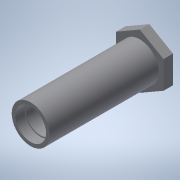
# Autodesk Inventor part: steering_stand_off_bush
Saved by Autodesk Inventor 2020 (Build 240168000, 168)
## iProperties
Created: 2015-12-06
Part Number: steering_stand_off_bush
Material: Genérico
Document SubType Name: Modeling
Designer: MIGUEL ANGEL
Density: 1 g/cm^3
Appearance: Valor por defecto
Author: MIGUEL ANGEL
Autodesk Inventor part; units mm, degrees
ref_plane "YZ Plane" through (0, 0, 0) normal (1, 0, 0) x (0, 1, 0)
ref_plane "XZ Plane" through (0, 0, 0) normal (0, 1, 0) x (-1, 0, 0)
ref_plane "XY Plane" through (0, 0, 0) normal (0, 0, 1) x (1, 0, 0)
sketch "Boceto1" plane through (0, 0, 0) normal (0, 1, 0) x (-1, 0, 0)
  circle A0 centre (0, 0) radius 8
  dimension "d0" = 16
  constraints: 1 centre point, 1 coincident
  measures "d0" diameter of A0
extrude "Extrusión1" add sketch "Boceto1" along normal blind 46
sketch "Boceto2" plane through (0, 46, 0) normal (0, 1, 0) x (1, 0, 0)
  line L0 (0, 11.547) -> (10, 5.7735)
  line L1 (10, 5.7735) -> (10, -5.7735)
  line L2 (10, -5.7735) -> (0, -11.547)
  line L3 (0, -11.547) -> (-10, -5.7735)
  line L4 (-10, -5.7735) -> (-10, 5.7735)
  line L5 (-10, 5.7735) -> (0, 11.547)
  point P0 (0, 0)
  point P1 (0, 0)
  point P2 (-10, 0)
  dimension "d3" = 10
  constraints: 12 end point, 1 coincident, 1 horizontal alignment, 1 midpoint, 13 other
  measures "d3" horizontal distance of L1.end L2.end
extrude "Extrusión2" add sketch "Boceto2" along normal blind 4
sketch "Boceto3" plane through (0, 0, 0) normal (0, -1, 0) x (1, 0, 0)
  circle A0 centre (0, 0) radius 8 projected
  circle A1 centre (0, 0) radius 6
  dimension "d6" = 2
  constraints: 1 centre point
  measures "d6" radial gap between concentric circles of A0 A1
extrude "Extrusión3" cut sketch "Boceto3" against normal through all contours A1
sketch "Boceto4" plane through (0, 0, 0) normal (0, 0, 1) x (1, 0, 0)
  line L0 (-6, 0) -> (-6, 50) projected
  line L1 (6, 0) -> (6, 50) projected
  line L2 (-6, 0) -> (-6.5, 0)
  line L3 (-8, 0) -> (8, 0) projected
  line L4 (-6.5, 4) -> (-6.5, 0)
  line L5 (-6.5, 4) -> (-6, 4)
  line L6 (-6.5, 0) -> (-6, 0)
  line L7 (0, -14.3469) -> (0, 54.7161)
  line L8 (-6.5, 50) -> (-6.5, 46)
  line L9 (-6.5, 46) -> (-6, 46)
  line L10 (-10, 50) -> (0, 50) projected
  point P0 (0, 0)
  dimension "d9" = 0.5
  dimension "d10" = 4
  dimension "d11" = 0.5
  dimension "d12" = 4
  constraints: 14 end point, 4 point on line, 2 perpendicular, 2 vertical, 1 collinear, 1 parallel
  measures "d9" distance of L0.start L2.end
  measures "d10" distance of L4.start L2.end
  measures "d11" distance of L8.end L9.end
  measures "d12" distance of L8.start L8.end
revolve "Revolución1" cut sketch "Boceto4" angle 360 about axis through (0, -14.3469, 0) along (0, 1, 0) contours L2 L4 L5 L0 | L9 L8 L10 L0
